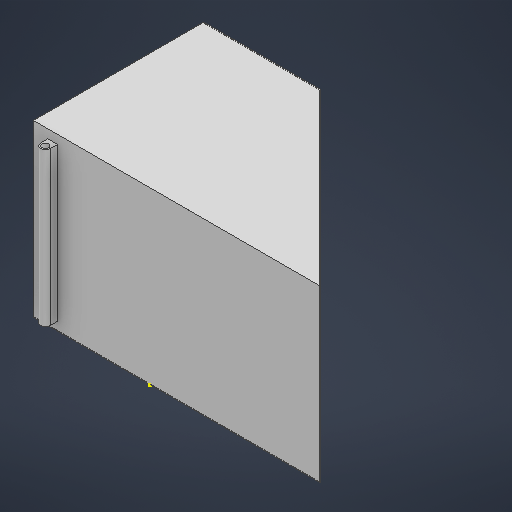
# Autodesk Inventor part: Cajon_ascensor_mejorsita
Saved by Autodesk Inventor 2026.2 (Build 302298010, 298A)
## iProperties
Created: 2026-04-28
Part Number: Cajon_ascensor_mejorsita
Material: Genérico
Document SubType Name: Modeling
Designer: agusb
Density: 1 g/cm^3
Appearance: Valor por defecto
Author: agusb
Autodesk Inventor part; units mm, degrees
ref_plane "YZ Plane" through (0, 0, 0) normal (1, 0, 0) x (0, 1, 0)
ref_plane "XZ Plane" through (0, 0, 0) normal (0, 1, 0) x (-1, 0, 0)
ref_plane "XY Plane" through (0, 0, 0) normal (0, 0, 1) x (1, 0, 0)
sketch "Boceto1" plane through (0, 0, 0) normal (0, 1, 0) x (-1, 0, 0)
  line L0 (0, 0) -> (0, -350)
  line L1 (0, -350) -> (-350, 0)
  line L2 (-350, 0) -> (0, 0)
  dimension "d0" = 350
  dimension "d1" = 45
  constraints: 6 end point, 1 perpendicular, 1 vertical
  measures "d0" distance of L0.start L0.end
  measures "d1" angle of L0 L1
extrude "Extrusión1" add sketch "Boceto1" along normal blind 1
sketch "Boceto2" plane through (0, 1, 0) normal (0, 1, 0) x (1, 0, 0)
  line L0 (350, 0) -> (0, 350) projected
  line L1 (174.2929, 174.2929) -> (348.5858, 0)
  line L2 (0, 0) -> (350, 0) projected
  line L3 (174.2929, 174.2929) -> (420.7803, 174.2929) construction
  line L4 (348.5858, 1) -> (-0.0002, 1)
  line L5 (0, 350) -> (0, 0) projected
  line L6 (174.2929, 174.2929) -> (0, 348.5858)
  point P0 (347.5858, 1)
  point P1 (0, 1)
  dimension "d5" = 45
  dimension "d6" = 1
  dimension "d7" = 348.586
  constraints: 8 end point, 3 point on line, 1 equal length, 1 horizontal, 1 perpendicular
  measures "d5" angle of L1 L3
  measures "d6" distance of L1.end L4.start
  measures "d7" distance of L4.start L4.end
extrude "Extrusión2" add sketch "Boceto2" along normal blind 348 contours L2 L1 L6 L5 L0 | L2 L5 L4 L1
sketch "Boceto3" plane through (0, 349, 0) normal (0, 1, 0) x (1, 0, 0)
  line L0 (0, 350) -> (0, 0) projected
  line L1 (0, 0) -> (0, 350)
  line L2 (0, 0) -> (350, 0) projected
  line L3 (0, 350) -> (350, 0)
  line L4 (350, 0) -> (0, 0)
  constraints: 6 end point, 1 perpendicular, 1 vertical
extrude "Extrusión3" add sketch "Boceto3" along normal blind 1
sketch "Boceto4" plane through (0, 0, -350) normal (-1, 0, 0) x (0, 0, 1)
  point P0 (350, 0)
sketch "Boceto5" plane through (0, 0, -350) normal (-1, 0, 0) x (0, 0, 1)
  line L0 (0, 0) -> (0, 350) projected
  line L1 (350, 0) -> (0, 0)
  line L2 (0, 0) -> (0, 350)
  line L3 (0, 350) -> (350, 350)
  line L4 (350, 350) -> (350, 0)
  line L5 (349, 1) -> (1.4142, 1) projected
  line L6 (1.4142, 1) -> (1.4142, 349) projected
  line L7 (349, 1) -> (1.4142, 1)
  line L8 (1.4142, 1) -> (1.4142, 349)
  line L9 (1.4142, 349) -> (349, 349)
  line L10 (349, 349) -> (349, 1)
  constraints: 16 end point, 4 parallel, 2 horizontal, 2 perpendicular
extrude "Extrusión4" add sketch "Boceto5" along normal blind 240
sketch "Boceto6" plane through (350, 0, 0) normal (0, 0, 1) x (1, 0, 0)
  line L0 (-590, 0) -> (-590, 350) projected
  line L1 (-590, 350) -> (-560, 350)
  line L2 (-350, 349) -> (-590, 349) projected
  line L3 (-590, 350) -> (-560, 350) construction
  line L4 (-560, 350) -> (-560, 332.3)
  line L5 (-590, 0) -> (-560, 0)
  line L6 (-350, 1) -> (-590, 1) projected
  line L7 (-590, 0) -> (-560, 0) construction
  line L8 (-560, 0) -> (-560, 17.7)
  line L9 (-560, 332.3) -> (-540, 332.3)
  line L10 (-540, 332.3) -> (-540, 17.7)
  line L11 (-540, 17.7) -> (-560, 17.7)
  line L12 (-560, 17.7) -> (-560, 332.3)
  point P0 (-350, 0)
  dimension "d15" = 30
  dimension "d16" = 0
  dimension "d17" = 17.7
  dimension "d18" = 30
  dimension "d19" = 0
  dimension "d20" = 17.7
  dimension "d21" = 90
  dimension "d22" = 20
  constraints: 20 end point, 4 parallel, 3 horizontal, 3 perpendicular, 2 collinear
  measures "d15" distance of L0.end L1.end
  measures "d16" distance between parallel lines of L1 L3
  measures "d17" distance of L1.end L4.end
  measures "d18" distance of L0.start L5.end
  measures "d19" distance between parallel lines of L5 L7
  measures "d20" distance of L5.end L8.end
  measures "d21" angle of L8 L5
  measures "d22" distance of L10.end L11.end
extrude "Extrusión5" add sketch "Boceto6" along normal blind 25 contours L12 L9 L10 L11
fillet "Empalme1" radius 10 2 edges at (-210, 175, 25) (-190, 175, 25)
sketch "Boceto8" plane through (-210, 332.3, 0) normal (0, 1, 0) x (1, 0, 0)
  line L0 (0, 0) -> (0, -15) projected
  line L1 (0, -15) -> (10, -15)
  circle A0 centre (10, -15) radius 7
  point P0 (210, 0)
  dimension "d29" = 10
  dimension "d30" = 14
  constraints: 2 end point, 1 centre point, 1 coincident, 1 horizontal
  measures "d29" distance of L0.end L1.end
  measures "d30" diameter of A0
extrude "Extrusión7" cut sketch "Boceto8" against normal blind 1000
